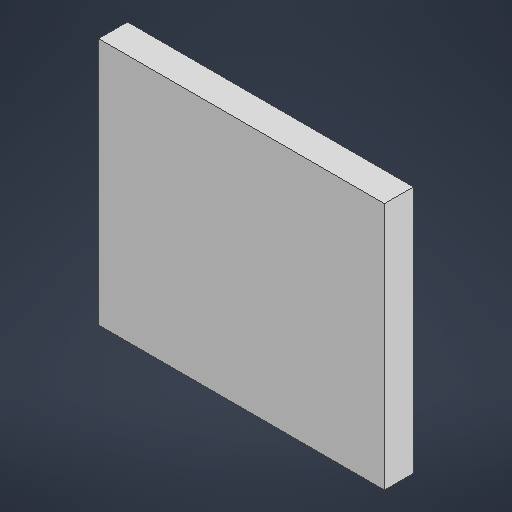
# Autodesk Inventor part: 垃圾
Saved by Autodesk Inventor 2025 (Build 290162000, 162)
## iProperties
Created: 2026-01-24
Part Number: 垃圾
Material: 常规
Document SubType Name: Modeling
Designer: XH
Density: 1 g/cm^3
Appearance: 默认
Author: XH
Autodesk Inventor part; units mm, degrees
ref_plane "YZ Plane" through (0, 0, 0) normal (1, 0, 0) x (0, 1, 0)
ref_plane "XZ Plane" through (0, 0, 0) normal (0, 1, 0) x (-1, 0, 0)
ref_plane "XY Plane" through (0, 0, 0) normal (0, 0, 1) x (1, 0, 0)
sketch "草图1" plane through (0, 0, 0) normal (0, 0, 1) x (1, 0, 0)
  line L0 (14.8148, -12.8571) -> (-14.8148, -12.8571)
  line L1 (-14.8148, -12.8571) -> (-14.8148, 12.8571)
  line L2 (-14.8148, 12.8571) -> (14.8148, 12.8571)
  line L3 (14.8148, 12.8571) -> (14.8148, -12.8571)
  line L4 (14.8148, -12.8571) -> (-14.8148, 12.8571) construction
  line L5 (-14.8148, -12.8571) -> (14.8148, 12.8571) construction
  point P0 (0, 0)
  constraints: 12 end point, 2 midpoint, 2 parallel, 1 horizontal, 1 perpendicular
extrude "拉伸1" add sketch "草图1" along normal blind 3
